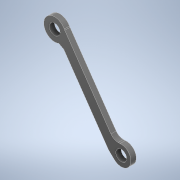
# Autodesk Inventor part: Pieza9
Saved by Autodesk Inventor 2022 (Build 260153000, 153)
## iProperties
Created: 2022-11-04
Part Number: Pieza9
Material: Resina acetálica, negra
Document SubType Name: Modeling
Designer: Mauricio Guerrero
Density: 1.425 g/cm^3
Appearance: Suave - Negro
Author: Mauricio Guerrero
## iProperties of the stored document Pieza9_3DPrint.ipt
Created: 2022-11-06
Part Number: Pieza9_3DPrint
Material: Genérico
Document SubType Name: Modeling
Designer: Mauricio Guerrero
Density: 1 g/cm^3
Appearance: Valor por defecto
Author: Mauricio Guerrero
Autodesk Inventor part; units mm, degrees
ref_plane "YZ Plane" through (0, 0, 0) normal (1, 0, 0) x (0, 1, 0)
ref_plane "XZ Plane" through (0, 0, 0) normal (0, 1, 0) x (-1, 0, 0)
ref_plane "XY Plane" through (0, 0, 0) normal (0, 0, 1) x (1, 0, 0)
sketch "Boceto1" plane through (0, 0, 0) normal (0, 0, 1) x (1, 0, 0)
  circle A0 centre (690.2291, 250.8095) radius 1.25
  arc A1 (692.4377, 251.981) -> (691.1952, 248.5037) centre (690.2291, 250.8095) ccw
  circle A2 centre (705.5291, 233.3595) radius 1.25
  line L0 (692.5597, 251.7803) -> (703.1648, 236.452)
  line L1 (692.3398, 247.8801) -> (702.5235, 233.1607)
  arc A3 (702.665, 232.951) -> (702.6433, 232.9876) centre (702.3966, 232.8169) ccw
  arc A4 (703.9859, 231.7221) -> (705.2332, 235.59) centre (705.5291, 233.3595) ccw
  line L2 (702.7965, 232.8432) -> (703.9859, 231.7221)
  line L3 (704.8095, 235.59) -> (705.2332, 235.59)
  arc A5 (703.1648, 236.452) -> (704.8095, 235.59) centre (704.8095, 237.59) ccw
  arc A6 (702.5235, 233.1607) -> (702.7965, 232.8432) centre (704.1683, 234.2986) ccw
  line L4 (692.3398, 247.8801) -> (691.1952, 248.5037)
  arc A7 (692.4377, 251.981) -> (692.5597, 251.7803) centre (694.2045, 252.9182) ccw
  point P0 (0, 0)
  dimension "d7" = 2.5
  dimension "d8" = 5
  dimension "d9" = 2.5
  dimension "d11" = 15.3
  dimension "d12" = 17.45
  dimension "d18" = 4.5
  dimension "d19" = 2
  dimension "d20" = 2.4
  dimension "d21" = 2
  constraints: 12 point on circle, 10 end point, 8 centre point, 8 tangent, 2 coincident, 2 point on line, 1 equal radius, 1 horizontal, 1 parallel
  measures "d7" diameter of A0
  measures "d8" diameter of A1
  measures "d9" diameter of A2
  measures "d11" horizontal distance of A2.centre A0.centre
  measures "d12" vertical distance of A2.centre A0.centre
  measures "d18" diameter of A4
  measures "d19" radius of A5
  measures "d20" distance between parallel lines of L0 L1
  measures "d21" radius of A7
extrude "Extrusión1" add sketch "Boceto1" along normal blind 1.2
